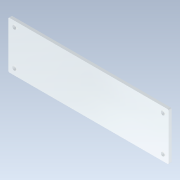
# Autodesk Inventor part: HeightPlates
Saved by Autodesk Inventor 2022.2 (Build 262287000, 287)
## iProperties
Created: 2021-12-01
Part Number: HeightPlates
Material: Generic
Document SubType Name: Modeling
Designer: Fabijan_Sven
Density: 1 g/cm^3
Appearance: Clear
Author: Fabijan_Sven
Autodesk Inventor part; units mm, degrees
ref_plane "YZ Plane" through (0, 0, 0) normal (1, 0, 0) x (0, 1, 0)
ref_plane "XZ Plane" through (0, 0, 0) normal (0, 1, 0) x (-1, 0, 0)
ref_plane "XY Plane" through (0, 0, 0) normal (0, 0, 1) x (1, 0, 0)
sketch "Sketch1" plane through (0, 0, 0) normal (0, 0, 1) x (1, 0, 0)
  line L0 (0, 0) -> (270, 0)
  line L1 (270, 0) -> (270, 80)
  line L2 (270, 80) -> (0, 80)
  line L3 (0, 80) -> (0, 0)
  dimension "d2" = 80
  dimension "d3" = 270
  constraints: 8 end point, 2 parallel, 1 horizontal, 1 perpendicular
  measures "d2" distance of L0.end L1.end
  measures "d3" distance of L1.end L2.end
extrude "Extrusion1" add sketch "Sketch1" along normal blind 5
sketch "Sketch2" plane through (0, 0, 5) normal (0, 0, 1) x (1, 0, 0)
  circle A0 centre (10, 70) radius 2.75
  circle A1 centre (260, 70) radius 2.75
  circle A2 centre (260, 10) radius 2.75
  circle A3 centre (10, 10) radius 2.75
  line L0 (270, 80) -> (0, 80) projected
  line L1 (0, 80) -> (0, 0) projected
  line L2 (270, 0) -> (270, 80) projected
  line L3 (0, 0) -> (270, 0) projected
  dimension "d4" = 10
  dimension "d5" = 10
  dimension "d6" = 10
  dimension "d7" = 10
  dimension "d8" = 10
  dimension "d9" = 10
  dimension "d10" = 10
  dimension "d11" = 10
  dimension "d12" = 5.5
  dimension "d13" = 5.5
  dimension "d14" = 5.5
  dimension "d15" = 5.5
  constraints: 4 centre point
  measures "d4" distance from line of L0 A0.centre
  measures "d5" distance from line of L1 A0.centre
  measures "d6" distance from line of L0 A1.centre
  measures "d7" distance from line of L2 A1.centre
  measures "d8" distance from line of L2 A2.centre
  measures "d9" distance from line of L3 A2.centre
  measures "d10" distance from line of L3 A3.centre
  measures "d11" distance from line of L1 A3.centre
  measures "d12" diameter of A0
  measures "d13" diameter of A1
  measures "d14" diameter of A2
  measures "d15" diameter of A3
hole "Hole1" at (10, 70, 5) at (10, 10, 5) at (260, 10, 5) at (260, 70, 5) direction (0, 0, -1) diameter 5.5 end through all
fillet "Fillet1" radius 2 4 edges at (0, 80, 2.5) (270, 80, 2.5) (270, 0, 2.5) (0, 0, 2.5)
equation "\"d5\" = d4"
equation "\"d6\" = d4"
equation "\"d7\" = d4"
equation "\"d8\" = d4"
equation "\"d9\" = d4"
equation "\"d10\" = d4"
equation "\"d11\" = d4"
equation "\"d13\" = d12"
equation "\"d14\" = d12"
equation "\"d15\" = d12"
equation "\"d16\" = d12"
body "Solid1"
